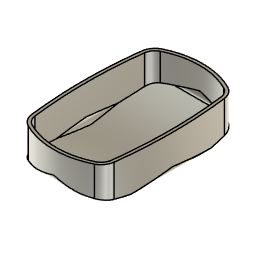
26 (Autodesk Fusion 360 design; units mm, degrees)
Autodesk Fusion 360 part; units mm, degrees
note: some values were not read from the file. Chosen so that the rebuilt part matches the saved one: which pieces of a blend or face edit are solid.
sketch "草图1" plane through (0, 0, 0) normal (1, 0, 0) x (0, 1, 0)
  line L0 (-50, 25) -> (-50, 10.1282)
  line L1 (0, 75) -> (0, -75) construction
  line L2 (-50, 25) -> (50, 25)
  line L3 (50, 25) -> (50, 10.1282)
  arc A0 (-50, 10.1282) -> (-46.125, 5.2565) centre (-45, 10.1282) ccw
  arc A1 (-46.125, 5.2565) -> (46.125, 5.2565) centre (0, 205) ccw
  arc A2 (46.125, 5.2565) -> (50, 10.1282) centre (45, 10.1282) ccw
  arc A3 (45.675, 7.2052) -> (48, 10.1282) centre (45, 10.1282) ccw
  line L4 (48, 23) -> (48, 10.1282)
  line L5 (-48, 23) -> (48, 23)
  line L6 (-48, 23) -> (-48, 10.1282)
  arc A4 (-48, 10.1282) -> (-45.675, 7.2052) centre (-45, 10.1282) ccw
  arc A5 (-45.675, 7.2052) -> (45.675, 7.2052) centre (0, 205) ccw
  line L7 (-48, 23) -> (-48, 25)
  line L8 (48, 23) -> (48, 25)
  dimension "d1" = 100
  dimension "d2" = 5
  dimension "d3" = 205
  dimension "d4" = 25
  dimension "d20" = 2
  constraint vertical L0
  constraint vertical L1
  constraint perpendicular L0 L2
  constraint perpendicular L2 L3
  constraint tangent L0 A0
  constraint tangent L3 A2
  constraint symmetric L0 L1 L3
  constraint symmetric L1 A0.centre A2.centre
  constraint symmetric L1 A0.end A1.end
  constraint tangent A1 A2
  constraint midpoint A1 origin
  constraint coincident L2 L7.end
  constraint perpendicular L2 L7
  constraint coincident L2 L8.end
  constraint perpendicular L2 L8
  measures "d1" distance of L0.start L2.end
  measures "d2" radius of A2
  measures "d3" radius of A1
  measures "d4" distance of L2 origin
extrude "拉伸1" add sketch "草图1" along normal mid plane 60 makes body 1
sketch "草图2" plane through (0, 0, 25) normal (0, 0, 1) x (-1, 0, 0)
  line L0 (30, 50) -> (-30, 50)
  line L1 (-30, 50) -> (-30, -50)
  line L2 (-30, -50) -> (30, -50)
  line L3 (30, -50) -> (30, 50)
  line L4 (60, 0) -> (-100, 0) construction
  line L5 (0, -75) -> (0, 75) construction
  arc A0 (-22.2222, -44.7903) -> (22.2222, -44.7903) centre (0, 0) ccw
  arc A1 (22.2222, 44.7903) -> (-22.2222, 44.7903) centre (0, 0) ccw
  arc A2 (22.2222, -44.7903) -> (27.7011, -37.0679) centre (17.7778, -35.8323) ccw
  arc A3 (-27.7011, -37.0679) -> (-22.2222, -44.7903) centre (-17.7778, -35.8323) ccw
  arc A4 (-22.2222, 44.7903) -> (-27.7011, 37.0679) centre (-17.7778, 35.8323) ccw
  arc A5 (27.7011, 37.0679) -> (22.2222, 44.7903) centre (17.7778, 35.8323) ccw
  arc A6 (27.7011, -37.0679) -> (27.7011, 37.0679) centre (-270, 0) ccw
  arc A7 (-27.7011, 37.0679) -> (-27.7011, -37.0679) centre (270, 0) ccw
  arc A8 (25.7165, -36.8207) -> (25.7165, 36.8207) centre (-270, 0) ccw
  arc A9 (25.7165, 36.8207) -> (21.3333, 42.9987) centre (17.7778, 35.8323) ccw
  arc A10 (21.3333, 42.9987) -> (-21.3333, 42.9987) centre (0, 0) ccw
  arc A11 (-21.3333, 42.9987) -> (-25.7165, 36.8207) centre (-17.7778, 35.8323) ccw
  arc A12 (-25.7165, 36.8207) -> (-25.7165, -36.8207) centre (270, 0) ccw
  arc A13 (-25.7165, -36.8207) -> (-21.3333, -42.9987) centre (-17.7778, -35.8323) ccw
  arc A14 (-21.3333, -42.9987) -> (21.3333, -42.9987) centre (0, 0) ccw
  arc A15 (21.3333, -42.9987) -> (25.7165, -36.8207) centre (17.7778, -35.8323) ccw
  point P0 (0, -50)
  point P1 (0, 50)
  point P2 (30, 0)
  point P3 (-30, 0)
  dimension "d7" = 50
  dimension "d8" = 100
  dimension "d9" = 10
  dimension "d10" = 300
  dimension "d11" = 60
  dimension "d26" = -2
  constraint horizontal L4
  constraint vertical L5
  constraint symmetric L4 A0.start A1.end
  constraint symmetric L4 A0.end A1.start
  constraint symmetric L5 A0.end A0.start
  constraint midpoint A0 P0
  constraint midpoint A1 P1
  constraint symmetric L4 A0 A1
  constraint symmetric L4 A3.start A4.end
  constraint symmetric L4 A2.end A5.start
  constraint symmetric L5 A2.end A3.start
  constraint equal A2 A3
  constraint equal A3 A4
  constraint equal A2 A5
  constraint tangent A0 A3
  constraint tangent A0 A2
  constraint tangent A1 A5
  constraint tangent A1 A4
  constraint tangent A5 A6
  constraint equal A6 A7
  constraint tangent A2 A6
  constraint midpoint A6 P2
  constraint midpoint A7 P3
  measures "d7" radius of A0
  measures "d8" distance of P0 P1
  measures "d9" radius of A3
  measures "d10" radius of A7
  measures "d11" distance of P2 P3
copy_body "复制和粘贴实体1" bodies 1 makes body 2
move_body "移动1" bodies 2 to x (-1, 0, 0) y (0, 1, 0) z (0, 0, -1) at (116.6799, 0, 20.2565)
move_body "移动2" bodies 2 to x (1, 0, 0) y (0, 1, 0) z (0, 0, 1) at (-116.6799, 0, 29.7435)
extrude "拉伸2" cut sketch "草图2" along normal mid plane 120 contours A0 A1 A2 A3 A4 A5 A6 A7 | A8 A9 A10 A11 A12 A13 A14 A15 keep common part bodies 1 2
sketch "草图3" plane through (0, 0, 0) normal (0, 1, 0) x (1, 0, 0)
  line L0 (-30, -45) -> (-30, -5)
  arc A0 (-25, 0) -> (-30, -5) centre (-25, -5) ccw
  line L1 (-25, 0) -> (25, 0)
  line L2 (-25, -50) -> (25, -50)
  line L3 (30, -45) -> (30, -5)
  arc A1 (25, -50) -> (30, -45) centre (25, -45) ccw
  arc A2 (30, -5) -> (25, 0) centre (25, -5) ccw
  arc A3 (-30, -45) -> (-25, -50) centre (-25, -45) ccw
  line L4 (-40, 0) -> (60, 0) construction
  line L5 (-40, -25) -> (60, -25) construction
  line L6 (0, 15) -> (0, -75) construction
  line L7 (28, -45) -> (28, -5)
  arc A4 (28, -5) -> (25, -2) centre (25, -5) ccw
  line L8 (-25, -2) -> (25, -2)
  arc A5 (-25, -2) -> (-28, -5) centre (-25, -5) ccw
  line L9 (-28, -45) -> (-28, -5)
  arc A6 (-28, -45) -> (-25, -48) centre (-25, -45) ccw
  line L10 (-25, -48) -> (25, -48)
  arc A7 (25, -48) -> (28, -45) centre (25, -45) ccw
  dimension "d14" = 25
  dimension "d15" = 5
  dimension "d16" = 60
  dimension "d23" = -2
  constraint tangent L0 A0
  constraint perpendicular L0 L1
  constraint horizontal L2
  constraint vertical L3
  constraint tangent L2 A1
  constraint horizontal L4
  constraint horizontal L5
  constraint collinear L1 L4
  constraint perpendicular L2 L6
  constraint symmetric L0 L3 L6
  constraint equal A1 A3
  constraint equal A0 A2
  constraint equal A0 A3
  constraint tangent L2 A3
  constraint tangent A0 L1
  constraint tangent L3 A2
  constraint tangent A2 L4
  constraint tangent L3 A1
  constraint symmetric L1 L2 L5
  constraint tangent L0 A3
  measures "d14" distance of L4 L5
  measures "d15" radius of A1
  measures "d16" distance of L0 L3
extrude "拉伸3" cut sketch "草图3" along normal mid plane 170 contours L0 A0 L1 L2 L3 A1 A2 A3 | L7 A4 L8 A5 L9 A6 L10 A7 keep common part bodies 1 2
combine "合并1" operation add target body 1 tool bodies 2
shell "抽壳1" thickness 2 removed faces 0 bodies 1
delete_body "移除实体1" bodies 3
extrude "拉伸4" add sketch "草图1" along normal mid plane 60 separate body contours L2 L5 L7 L8 | A3 L4 L5 L6 A4 A5 makes body 4
copy_body "复制和粘贴实体2" bodies 4 makes body 5
move_body "移动3" bodies 5 to x (1, 0, 0) y (0, 1, 0) z (0, 0, 1) at (120, 0, 0)
move_body "移动4" bodies 5 to x (-1, 0, 0) y (0, 1, 0) z (0, 0, -1) at (228.933, 0, 50)
move_body "移动5" bodies 5 to x (1, 0, 0) y (0, 1, 0) z (0, 0, 1) at (-108.933, 0, 0)
combine "合并2" operation add target body 4 tool bodies 5
extrude "拉伸5" cut sketch "草图3" along normal mid plane 174 contours L7 A4 L8 A5 L9 A6 L10 A7 keep common part bodies 4
extrude "拉伸6" cut sketch "草图2" along normal mid plane 72 contours A8 A9 A10 A11 A12 A13 A14 A15 keep common part bodies 4
combine "合并3" operation cut target body 1 tool bodies 4
sketch "草图4" plane through (0, 0, 0) normal (0, 1, 0) x (1, 0, 0)
  line L0 (-30, -50) -> (30, -50)
  line L1 (30, -50) -> (30, -25)
  line L2 (30, -25) -> (-30, -25)
  line L3 (-30, -25) -> (-30, -50)
  line L4 (-50, 0) -> (45, 0) construction
  line L5 (0, -70) -> (0, 16) construction
  dimension "d29" = 25
  dimension "d30" = 25
  dimension "d31" = 60
  constraint horizontal L0
  constraint vertical L1
  constraint horizontal L2
  constraint vertical L3
  constraint horizontal L4
  constraint perpendicular L4 L5
  constraint symmetric L1 L3 L5
  measures "d29" distance of L0 L2
  measures "d30" distance of L2 L4
  measures "d31" distance of L1 L3
extrude "拉伸7" cut sketch "草图4" along normal mid plane 246 bodies 1
